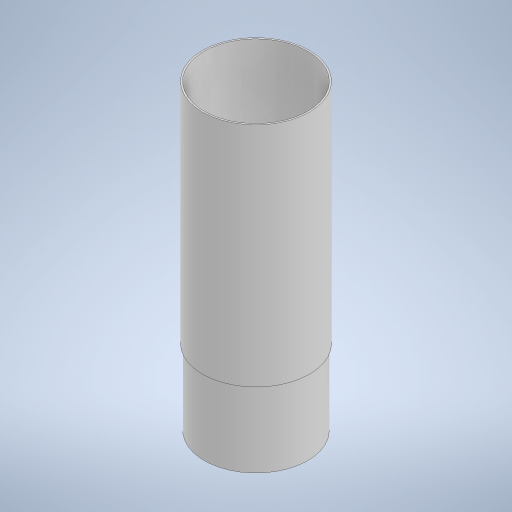
# Autodesk Inventor part: MidTube
Saved by Autodesk Inventor 2023.2 (Build 272271030, 271C)
## iProperties
Created: 2023-02-12
Part Number: MidTube
Material: Generic
Document SubType Name: Modeling
Designer: Lukas
Density: 1 g/cm^3
Appearance: Default
d6: 33.200 mm
d9: 200.000 mm
Author: Lukas
Autodesk Inventor part; units mm, degrees
ref_plane "YZ Plane" through (0, 0, 0) normal (1, 0, 0) x (0, 1, 0)
ref_plane "XZ Plane" through (0, 0, 0) normal (0, 1, 0) x (-1, 0, 0)
ref_plane "XY Plane" through (0, 0, 0) normal (0, 0, 1) x (1, 0, 0)
sketch "Sketch1" plane through (0, 0, 0) normal (1, 0, 0) x (0, 1, 0)
  line L0 (-100, -33.2) -> (50, -33.2)
  line L1 (50, -33.2) -> (50, -34.3)
  line L2 (-100, -34.2) -> (-100, -33.2)
  line L3 (100, -34.3) -> (100, -35.3)
  line L4 (100, -35.3) -> (-50, -35.3)
  line L5 (-140, 0) -> (140, 0) projected
  line L6 (100, -34.3) -> (50, -34.3)
  line L7 (-100, -34.2) -> (-50, -34.2)
  line L8 (-50, -34.2) -> (-50, -35.3)
  point P0 (0, 0)
  point P1 (-100, -33.875)
  point P2 (100, -34.75)
  dimension "d6" = 33.2
  dimension "d7" = 50
  dimension "d9" = 200
  dimension "d13" = 2.1
  dimension "d16" = 100
  dimension "d26" = 1
  dimension "d27" = 1
  dimension "d28" = 34.3
  dimension "d29" = 34.2
  constraints: 16 end point, 2 horizontal, 2 parallel, 2 point on line, 2 vertical
  measures "d6" distance from line of point (0, 0) L0
  measures "d7" distance of L1.end L3.start
  measures "d9" distance from line of point (100, -34.75) L2
  measures "d13" distance between parallel lines of L4 L0
  measures "d16" distance from line of point (0, 0) L3
  measures "d26" distance between parallel lines of L6 L4
  measures "d27" distance between parallel lines of L7 L0
  measures "d28" distance between parallel lines of L6 L5
  measures "d29" distance between parallel lines of L5 L7
revolve "Revolution1" add sketch "Sketch1" angle 360 about axis through (0, -10, 0) along (0, 1, 0)
sketch "Sketch2" plane through (0, 0, 0) normal (1, 0, 0) x (0, 1, 0)
  line L0 (71, 3) -> (65, 3)
  line L1 (65, 3) -> (65, -3)
  line L2 (65, -3) -> (71, -3)
  line L3 (71, -3) -> (71, 3)
  line L4 (100, -35.3) -> (100, 35.3) projected
  point P0 (0, 0)
  dimension "d17" = 3
  dimension "d18" = 3
  dimension "d19" = 6
  dimension "d20" = 29
  constraints: 8 end point, 2 parallel, 1 horizontal, 1 perpendicular
  measures "d17" distance from line of point (0, 0) L0
  measures "d18" distance from line of point (0, 0) L2
  measures "d19" distance between parallel lines of L3 L1
  measures "d20" distance between parallel lines of L4 L3
extrude "Extrusion1" [suppressed]
equation "\"d16\" = 0.5 * d9"
equation "\"gap\" = 0.1"
body "Solid1"
